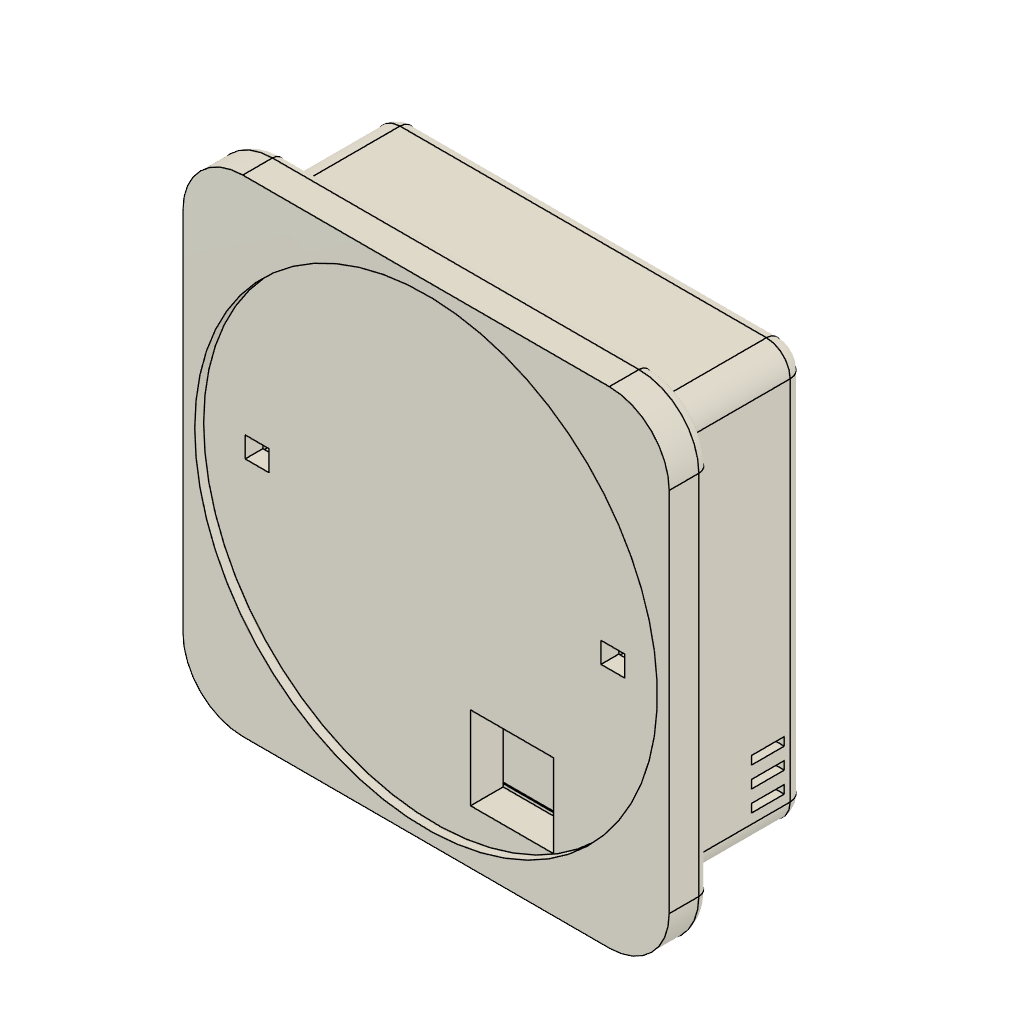
co2_wall_sensor (Autodesk Fusion 360 design; units mm, degrees)
part number: 2026-10-04-22-38-18-043
part number: 2026-10-04-22-38-18-293
part number: 2026-10-04-22-38-22-354
part number: 2026-10-04-22-38-25-106
part number: 2026-10-04-22-38-27-455
part number: 2026-10-04-22-38-30-527
part number: 2026-10-04-22-38-34-110
part number: 2026-10-04-22-38-35-616
part number: 2026-10-04-22-38-36-232
Autodesk Fusion 360 part; units mm, degrees
ref_plane "Arbeitsebene1" through (0, 0, 11) normal (0, 0, 1) x (1, 0, 0) in component "Housing"
sketch "Skizze1" plane through (0, 0, 11) normal (0, 0, 1) x (1, 0, 0) in component "Housing"
  line L0 (-34.9, -34.9) -> (34.9, -34.9)
  line L1 (34.9, -34.9) -> (34.9, 34.9)
  line L2 (34.9, 34.9) -> (-34.9, 34.9)
  line L3 (-34.9, 34.9) -> (-34.9, -34.9)
extrude "BaseBody (1)" add sketch "Skizze1" along normal mid plane 22 makes body 1 in component "Housing"
fillet "CornerRadius" radius 4 4 edges at (-34.9, 34.9, 11) (34.9, 34.9, 11) (34.9, -34.9, 11) (-34.9, -34.9, 11) on bodies 1 in component "Housing"
fillet "SoftFrontEdge" radius 2.5 64 edges at (-33.7284, -33.7284, 0) (0, -34.9, 0) (33.7284, -33.7284, 0) (34.9, 0, 0) (33.7284, 33.7284, 0) (0, 34.9, 0) (-33.7284, 33.7284, 0) (-34.9, 0, 0) (-34.9, 0, 0) (-33.7284, 33.7284, 0) (0, 34.9, 0) (33.7284, 33.7284, 0) (34.9, 0, 0) (33.7284, -33.7284, 0) (0, -34.9, 0) (-33.7284, -33.7284, 0) (-33.7284, 33.7284, 0) (-34.9, 0, 0) (-33.7284, -33.7284, 0) (0, -34.9, 0) (33.7284, -33.7284, 0) (34.9, 0, 0) (33.7284, 33.7284, 0) (0, 34.9, 0) (0, 34.9, 0) (33.7284, 33.7284, 0) (34.9, 0, 0) (33.7284, -33.7284, 0) (0, -34.9, 0) (-33.7284, -33.7284, 0) (-34.9, 0, 0) (-33.7284, 33.7284, 0) (33.7284, 33.7284, 0) (0, 34.9, 0) (-33.7284, 33.7284, 0) (-34.9, 0, 0) (-33.7284, -33.7284, 0) (0, -34.9, 0) (33.7284, -33.7284, 0) (34.9, 0, 0) (34.9, 0, 0) (33.7284, -33.7284, 0) (0, -34.9, 0) (-33.7284, -33.7284, 0) (-34.9, 0, 0) (-33.7284, 33.7284, 0) (0, 34.9, 0) (33.7284, 33.7284, 0) (33.7284, -33.7284, 0) (34.9, 0, 0) (33.7284, 33.7284, 0) (0, 34.9, 0) (-33.7284, 33.7284, 0) (-34.9, 0, 0) (-33.7284, -33.7284, 0) (0, -34.9, 0) (0, -34.9, 0) (-33.7284, -33.7284, 0) (-34.9, 0, 0) (-33.7284, 33.7284, 0) (0, 34.9, 0) (33.7284, 33.7284, 0) (34.9, 0, 0) (33.7284, -33.7284, 0) on bodies 1 in component "Housing"
ref_plane "Arbeitsebene2" through (0, 0, 21.25) normal (0, 0, 1) x (1, 0, 0) in component "Housing"
sketch "Skizze2" plane through (0, 0, 21.25) normal (0, 0, 1) x (1, 0, 0) in component "Housing"
  line L0 (-32.9, -32.9) -> (32.9, -32.9)
  line L1 (32.9, -32.9) -> (32.9, 32.9)
  line L2 (32.9, 32.9) -> (-32.9, 32.9)
  line L3 (-32.9, 32.9) -> (-32.9, -32.9)
extrude "CoverSeat (1)" cut sketch "Skizze2" along normal mid plane 3.5 bodies 1 in component "Housing"
ref_plane "Arbeitsebene3" through (0, 0, 11.25) normal (0, 0, 1) x (1, 0, 0) in component "Housing"
sketch "Skizze3" plane through (0, 0, 11.25) normal (0, 0, 1) x (1, 0, 0) in component "Housing"
  line L0 (-31.4, -7.7) -> (27.2, -7.7)
  line L1 (27.2, -7.7) -> (27.2, 27.9)
  line L2 (27.2, 27.9) -> (-31.4, 27.9)
  line L3 (-31.4, 27.9) -> (-31.4, -7.7)
extrude "DisplayBay (1)" cut sketch "Skizze3" along normal mid plane 18.5 bodies 1 in component "Housing"
ref_plane "Arbeitsebene4" through (0, 0, 0.75) normal (0, 0, 1) x (1, 0, 0) in component "Housing"
sketch "Skizze4" plane through (0, 0, 0.75) normal (0, 0, 1) x (1, 0, 0) in component "Housing"
  line L0 (-20.9, -5.7) -> (20.9, -5.7)
  line L1 (20.9, -5.7) -> (20.9, 25.9)
  line L2 (20.9, 25.9) -> (-20.9, 25.9)
  line L3 (-20.9, 25.9) -> (-20.9, -5.7)
extrude "DisplayWindow (1)" cut sketch "Skizze4" along normal mid plane 3.5 bodies 1 in component "Housing"
fillet "WindowCorners" radius 1 4 edges at (20.9, -5.7, 1) (-20.9, -5.7, 1) (-20.9, 25.9, 1) (20.9, 25.9, 1) on bodies 1 in component "Housing"
chamfer "WindowChamfer" distance 0.8 angle 45 8 edges at (0, 25.9, 0) (-20.6071, 25.6071, 0) (-20.9, 10.1, 0) (-20.6071, -5.4071, 0) (0, -5.7, 0) (20.6071, -5.4071, 0) (20.9, 10.1, 0) (20.6071, 25.6071, 0) tangent chain off on bodies 1 in component "Housing"
ref_plane "Arbeitsebene5" through (0, 0, 3.25) normal (0, 0, 1) x (1, 0, 0) in component "Housing"
sketch "Skizze5" plane through (0, 0, 3.25) normal (0, 0, 1) x (1, 0, 0) in component "Housing"
  circle A0 centre (-28.6, -4.9) radius 2.3
  circle A1 centre (-28.6, 25.1) radius 2.3
  circle A2 centre (24.4, -4.9) radius 2.3
  circle A3 centre (24.4, 25.1) radius 2.3
extrude "LcdBosses (1)" add sketch "Skizze5" along normal mid plane 2.5 bodies 1 in component "Housing"
ref_plane "Arbeitsebene6" through (0, 0, 2.85) normal (0, 0, 1) x (1, 0, 0) in component "Housing"
sketch "Skizze6" plane through (0, 0, 2.85) normal (0, 0, 1) x (1, 0, 0) in component "Housing"
  circle A0 centre (-28.6, -4.9) radius 1.5
  circle A1 centre (-28.6, 25.1) radius 1.5
  circle A2 centre (24.4, -4.9) radius 1.5
  circle A3 centre (24.4, 25.1) radius 1.5
extrude "M2InsertHoles (1)" cut sketch "Skizze6" along normal mid plane 3.5 bodies 1 in component "Housing"
ref_plane "Arbeitsebene7" through (0, 0, 11.25) normal (0, 0, 1) x (1, 0, 0) in component "Housing"
sketch "Skizze7" plane through (0, 0, 11.25) normal (0, 0, 1) x (1, 0, 0) in component "Housing"
  line L0 (-32.9, -32.9) -> (32.9, -32.9)
  line L1 (32.9, -32.9) -> (32.9, -10.2)
  line L2 (32.9, -10.2) -> (-32.9, -10.2)
  line L3 (-32.9, -10.2) -> (-32.9, -32.9)
extrude "Chin (1)" cut sketch "Skizze7" along normal mid plane 18.5 bodies 1 in component "Housing"
ref_plane "Arbeitsebene8" through (0, 0, 16.75) normal (0, 0, 1) x (1, 0, 0) in component "Housing"
sketch "Skizze8" plane through (0, 0, 16.75) normal (0, 0, 1) x (1, 0, 0) in component "Housing"
  line L0 (3, -10.7) -> (23, -10.7)
  line L1 (23, -10.7) -> (23, -7.2)
  line L2 (23, -7.2) -> (3, -7.2)
  line L3 (3, -7.2) -> (3, -10.7)
extrude "EspPassage (1)" cut sketch "Skizze8" along normal mid plane 7.5 bodies 1 in component "Housing"
ref_plane "Arbeitsebene9" through (0, 0, 10.75) normal (0, 0, 1) x (1, 0, 0) in component "Housing"
sketch "Skizze9" plane through (0, 0, 10.75) normal (0, 0, 1) x (1, 0, 0) in component "Housing"
  circle A0 centre (-30.5, -30.5) radius 2.5
  circle A1 centre (30.5, -30.5) radius 2.5
extrude "CoverBossesBottom (1)" add sketch "Skizze9" along normal mid plane 17.5 bodies 1 in component "Housing"
ref_plane "Arbeitsebene10" through (0, 0, 6.5) normal (0, 0, 1) x (1, 0, 0) in component "Housing"
sketch "Skizze10" plane through (0, 0, 6.5) normal (0, 0, 1) x (1, 0, 0) in component "Housing"
  circle A0 centre (-30.5, -12.6) radius 2.5
  circle A1 centre (30.5, -12.6) radius 2.5
extrude "CarrierBosses (1)" add sketch "Skizze10" along normal mid plane 9 bodies 1 in component "Housing"
ref_plane "Arbeitsebene11" through (0, 0, 17.85) normal (0, 0, 1) x (1, 0, 0) in component "Housing"
sketch "Skizze11" plane through (0, 0, 17.85) normal (0, 0, 1) x (1, 0, 0) in component "Housing"
  circle A0 centre (-30.5, -30.5) radius 1.5
  circle A1 centre (30.5, -30.5) radius 1.5
  circle A2 centre (-20, 30.4) radius 1.5
  circle A3 centre (20, 30.4) radius 1.5
extrude "M2InsertHoles (2)" cut sketch "Skizze11" along normal mid plane 3.5 bodies 1 in component "Housing"
ref_plane "Arbeitsebene12" through (0, 0, 9.35) normal (0, 0, 1) x (1, 0, 0) in component "Housing"
sketch "Skizze12" plane through (0, 0, 9.35) normal (0, 0, 1) x (1, 0, 0) in component "Housing"
  circle A0 centre (-30.5, -12.6) radius 1.5
  circle A1 centre (30.5, -12.6) radius 1.5
extrude "M2InsertHoles (3)" cut sketch "Skizze12" along normal mid plane 3.5 bodies 1 in component "Housing"
ref_plane "Arbeitsebene13" through (0, 0, 10.25) normal (0, 0, 1) x (1, 0, 0) in component "Housing"
sketch "Skizze13" plane through (0, 0, 10.25) normal (0, 0, 1) x (1, 0, 0) in component "Housing"
  line L0 (-32.9, -32.9) -> (-31.7, -32.9)
  line L1 (-31.7, -32.9) -> (-31.7, -10.2)
  line L2 (-31.7, -10.2) -> (-32.9, -10.2)
  line L3 (-32.9, -10.2) -> (-32.9, -32.9)
extrude "CarrierLedge (1)" add sketch "Skizze13" along normal mid plane 1.5 bodies 1 in component "Housing"
ref_plane "Arbeitsebene14" through (0, 0, 10.25) normal (0, 0, 1) x (1, 0, 0) in component "Housing"
sketch "Skizze14" plane through (0, 0, 10.25) normal (0, 0, 1) x (1, 0, 0) in component "Housing"
  line L0 (31.7, -32.9) -> (32.9, -32.9)
  line L1 (32.9, -32.9) -> (32.9, -10.2)
  line L2 (32.9, -10.2) -> (31.7, -10.2)
  line L3 (31.7, -10.2) -> (31.7, -32.9)
extrude "CarrierLedge (2)" add sketch "Skizze14" along normal mid plane 1.5 bodies 1 in component "Housing"
ref_plane "Arbeitsebene15" through (0, -33.9, 0) normal (0, 1, 0) x (0, 0, 1) in component "Housing"
sketch "Skizze15" plane through (0, -33.9, 0) normal (0, 1, 0) x (1, 0, 0) in component "Housing"
  line L0 (-21.7, -3.5) -> (-20.3, -3.5)
  line L1 (-20.3, -3.5) -> (-20.3, -9)
  line L2 (-20.3, -9) -> (-21.7, -9)
  line L3 (-21.7, -9) -> (-21.7, -3.5)
  line L4 (-18.2, -3.5) -> (-16.8, -3.5)
  line L5 (-16.8, -3.5) -> (-16.8, -9)
  line L6 (-16.8, -9) -> (-18.2, -9)
  line L7 (-18.2, -9) -> (-18.2, -3.5)
  line L8 (-14.7, -3.5) -> (-13.3, -3.5)
  line L9 (-13.3, -3.5) -> (-13.3, -9)
  line L10 (-13.3, -9) -> (-14.7, -9)
  line L11 (-14.7, -9) -> (-14.7, -3.5)
  line L12 (-11.2, -3.5) -> (-9.8, -3.5)
  line L13 (-9.8, -3.5) -> (-9.8, -9)
  line L14 (-9.8, -9) -> (-11.2, -9)
  line L15 (-11.2, -9) -> (-11.2, -3.5)
  line L16 (-7.7, -3.5) -> (-6.3, -3.5)
  line L17 (-6.3, -3.5) -> (-6.3, -9)
  line L18 (-6.3, -9) -> (-7.7, -9)
  line L19 (-7.7, -9) -> (-7.7, -3.5)
  line L20 (-4.2, -3.5) -> (-2.8, -3.5)
  line L21 (-2.8, -3.5) -> (-2.8, -9)
  line L22 (-2.8, -9) -> (-4.2, -9)
  line L23 (-4.2, -9) -> (-4.2, -3.5)
  line L24 (-0.7, -3.5) -> (0.7, -3.5)
  line L25 (0.7, -3.5) -> (0.7, -9)
  line L26 (0.7, -9) -> (-0.7, -9)
  line L27 (-0.7, -9) -> (-0.7, -3.5)
  line L28 (2.8, -3.5) -> (4.2, -3.5)
  line L29 (4.2, -3.5) -> (4.2, -9)
  line L30 (4.2, -9) -> (2.8, -9)
  line L31 (2.8, -9) -> (2.8, -3.5)
  line L32 (6.3, -3.5) -> (7.7, -3.5)
  line L33 (7.7, -3.5) -> (7.7, -9)
  line L34 (7.7, -9) -> (6.3, -9)
  line L35 (6.3, -9) -> (6.3, -3.5)
  line L36 (9.8, -3.5) -> (11.2, -3.5)
  line L37 (11.2, -3.5) -> (11.2, -9)
  line L38 (11.2, -9) -> (9.8, -9)
  line L39 (9.8, -9) -> (9.8, -3.5)
  line L40 (13.3, -3.5) -> (14.7, -3.5)
  line L41 (14.7, -3.5) -> (14.7, -9)
  line L42 (14.7, -9) -> (13.3, -9)
  line L43 (13.3, -9) -> (13.3, -3.5)
  line L44 (16.8, -3.5) -> (18.2, -3.5)
  line L45 (18.2, -3.5) -> (18.2, -9)
  line L46 (18.2, -9) -> (16.8, -9)
  line L47 (16.8, -9) -> (16.8, -3.5)
  line L48 (20.3, -3.5) -> (21.7, -3.5)
  line L49 (21.7, -3.5) -> (21.7, -9)
  line L50 (21.7, -9) -> (20.3, -9)
  line L51 (20.3, -9) -> (20.3, -3.5)
extrude "BottomVents (1)" cut sketch "Skizze15" along normal mid plane 3 bodies 1 in component "Housing"
ref_plane "Arbeitsebene16" through (-33.9, 0, 0) normal (1, 0, 0) x (0, 1, 0) in component "Housing"
sketch "Skizze16" plane through (-33.9, 0, 0) normal (1, 0, 0) x (0, 0, -1) in component "Housing"
  line L0 (-3.5, -29.25) -> (-9, -29.25)
  line L1 (-9, -29.25) -> (-9, -27.85)
  line L2 (-9, -27.85) -> (-3.5, -27.85)
  line L3 (-3.5, -27.85) -> (-3.5, -29.25)
  line L4 (-3.5, -25.75) -> (-9, -25.75)
  line L5 (-9, -25.75) -> (-9, -24.35)
  line L6 (-9, -24.35) -> (-3.5, -24.35)
  line L7 (-3.5, -24.35) -> (-3.5, -25.75)
  line L8 (-3.5, -22.25) -> (-9, -22.25)
  line L9 (-9, -22.25) -> (-9, -20.85)
  line L10 (-9, -20.85) -> (-3.5, -20.85)
  line L11 (-3.5, -20.85) -> (-3.5, -22.25)
extrude "SideVents (1)" cut sketch "Skizze16" along normal mid plane 3 bodies 1 in component "Housing"
ref_plane "Arbeitsebene17" through (33.9, 0, 0) normal (1, 0, 0) x (0, 1, 0) in component "Housing"
sketch "Skizze17" plane through (33.9, 0, 0) normal (1, 0, 0) x (0, 0, -1) in component "Housing"
  line L0 (-3.5, -29.25) -> (-9, -29.25)
  line L1 (-9, -29.25) -> (-9, -27.85)
  line L2 (-9, -27.85) -> (-3.5, -27.85)
  line L3 (-3.5, -27.85) -> (-3.5, -29.25)
  line L4 (-3.5, -25.75) -> (-9, -25.75)
  line L5 (-9, -25.75) -> (-9, -24.35)
  line L6 (-9, -24.35) -> (-3.5, -24.35)
  line L7 (-3.5, -24.35) -> (-3.5, -25.75)
  line L8 (-3.5, -22.25) -> (-9, -22.25)
  line L9 (-9, -22.25) -> (-9, -20.85)
  line L10 (-9, -20.85) -> (-3.5, -20.85)
  line L11 (-3.5, -20.85) -> (-3.5, -22.25)
extrude "SideVents (2)" cut sketch "Skizze17" along normal mid plane 3 bodies 1 in component "Housing"
ref_plane "Arbeitsebene18" through (0, 0, 16.1) normal (0, 0, 1) x (1, 0, 0) in component "Housing"
sketch "Skizze18" plane through (0, 0, 16.1) normal (0, 0, 1) x (1, 0, 0) in component "Housing"
  line L0 (6.5, -35.9) -> (19.5, -35.9)
  line L1 (19.5, -35.9) -> (19.5, -32.8)
  line L2 (19.5, -32.8) -> (6.5, -32.8)
  line L3 (6.5, -32.8) -> (6.5, -35.9)
extrude "BottomCableOpening (1)" cut sketch "Skizze18" along normal mid plane 6.6 bodies 1 in component "Housing"
ref_plane "Arbeitsebene19" through (0, 0, 16.1) normal (0, 0, 1) x (1, 0, 0) in component "Housing"
sketch "Skizze19" plane through (0, 0, 16.1) normal (0, 0, 1) x (1, 0, 0) in component "Housing"
  line L0 (6.5, -34.9) -> (19.5, -34.9)
  line L1 (19.5, -34.9) -> (19.5, -34.3)
  line L2 (19.5, -34.3) -> (6.5, -34.3)
  line L3 (6.5, -34.3) -> (6.5, -34.9)
extrude "BottomKnockout (1)" add sketch "Skizze19" along normal mid plane 6.6 bodies 1 in component "Housing"
ref_plane "Arbeitsebene1" through (0, 0, 12) normal (0, 0, 1) x (1, 0, 0) in component "SensorCarrier"
sketch "Skizze1 (2)" plane through (0, 0, 12) normal (0, 0, 1) x (1, 0, 0) in component "SensorCarrier"
  line L0 (-32.7, -32.7) -> (32.7, -32.7)
  line L1 (32.7, -32.7) -> (32.7, -10.4)
  line L2 (32.7, -10.4) -> (-32.7, -10.4)
  line L3 (-32.7, -10.4) -> (-32.7, -32.7)
extrude "Carrier (1)" add sketch "Skizze1 (2)" along normal mid plane 2 separate body makes body 2 in component "SensorCarrier"
ref_plane "Arbeitsebene2" through (0, 0, 12) normal (0, 0, 1) x (1, 0, 0) in component "SensorCarrier"
sketch "Skizze2 (2)" plane through (0, 0, 12) normal (0, 0, 1) x (1, 0, 0) in component "SensorCarrier"
  line L0 (-33.3, -35.3) -> (-27.7, -35.3)
  line L1 (-27.7, -35.3) -> (-27.7, -27.7)
  line L2 (-27.7, -27.7) -> (-33.3, -27.7)
  line L3 (-33.3, -27.7) -> (-33.3, -35.3)
extrude "BossNotch (1)" cut sketch "Skizze2 (2)" along normal mid plane 4 bodies 2 in component "SensorCarrier"
ref_plane "Arbeitsebene3" through (0, 0, 12) normal (0, 0, 1) x (1, 0, 0) in component "SensorCarrier"
sketch "Skizze3 (2)" plane through (0, 0, 12) normal (0, 0, 1) x (1, 0, 0) in component "SensorCarrier"
  line L0 (27.7, -35.3) -> (33.3, -35.3)
  line L1 (33.3, -35.3) -> (33.3, -27.7)
  line L2 (33.3, -27.7) -> (27.7, -27.7)
  line L3 (27.7, -27.7) -> (27.7, -35.3)
extrude "BossNotch (2)" cut sketch "Skizze3 (2)" along normal mid plane 4 bodies 2 in component "SensorCarrier"
ref_plane "Arbeitsebene4" through (0, 0, 8.05) normal (0, 0, 1) x (1, 0, 0) in component "SensorCarrier"
sketch "Skizze4 (2)" plane through (0, 0, 8.05) normal (0, 0, 1) x (1, 0, 0) in component "SensorCarrier"
  circle A0 centre (-30.5, -12.6) radius 1.2
  circle A1 centre (30.5, -12.6) radius 1.2
extrude "M2Clearance (1)" cut sketch "Skizze4 (2)" along normal mid plane 10.1 bodies 2 in component "SensorCarrier"
ref_plane "Arbeitsebene5" through (0, 0, 10.25) normal (0, 0, 1) x (1, 0, 0) in component "SensorCarrier"
sketch "Skizze5 (2)" plane through (0, 0, 10.25) normal (0, 0, 1) x (1, 0, 0) in component "SensorCarrier"
  line L0 (-11.5, -31.85) -> (-10.3, -31.85)
  line L1 (-10.3, -31.85) -> (-10.3, -11.25)
  line L2 (-10.3, -11.25) -> (-11.5, -11.25)
  line L3 (-11.5, -11.25) -> (-11.5, -31.85)
extrude "ScdGuide (1)" add sketch "Skizze5 (2)" along normal mid plane 1.5 bodies 2 in component "SensorCarrier"
ref_plane "Arbeitsebene6" through (0, 0, 10.25) normal (0, 0, 1) x (1, 0, 0) in component "SensorCarrier"
sketch "Skizze6 (2)" plane through (0, 0, 10.25) normal (0, 0, 1) x (1, 0, 0) in component "SensorCarrier"
  line L0 (10.3, -31.85) -> (11.5, -31.85)
  line L1 (11.5, -31.85) -> (11.5, -11.25)
  line L2 (11.5, -11.25) -> (10.3, -11.25)
  line L3 (10.3, -11.25) -> (10.3, -31.85)
extrude "ScdGuide (2)" add sketch "Skizze6 (2)" along normal mid plane 1.5 bodies 2 in component "SensorCarrier"
ref_plane "Arbeitsebene7" through (0, 0, 12) normal (0, 0, 1) x (1, 0, 0) in component "SensorCarrier"
sketch "Skizze7 (2)" plane through (0, 0, 12) normal (0, 0, 1) x (1, 0, 0) in component "SensorCarrier"
  line L0 (-16, -14.2) -> (-12, -14.2)
  line L1 (-12, -14.2) -> (-12, -10.1)
  line L2 (-12, -10.1) -> (-16, -10.1)
  line L3 (-16, -10.1) -> (-16, -14.2)
extrude "ScdCableNotch (1)" cut sketch "Skizze7 (2)" along normal mid plane 3 bodies 2 in component "SensorCarrier"
ref_plane "Arbeitsebene8" through (0, 0, 13.25) normal (0, 0, 1) x (1, 0, 0) in component "SensorCarrier"
sketch "Skizze8 (2)" plane through (0, 0, 13.25) normal (0, 0, 1) x (1, 0, 0) in component "SensorCarrier"
  line L0 (6.25, -19.9) -> (7.75, -19.9)
  line L1 (7.75, -19.9) -> (7.75, -10.4)
  line L2 (7.75, -10.4) -> (6.25, -10.4)
  line L3 (6.25, -10.4) -> (6.25, -19.9)
extrude "C3Rib (1)" add sketch "Skizze8 (2)" along normal mid plane 0.5 bodies 2 in component "SensorCarrier"
ref_plane "Arbeitsebene9" through (0, 0, 13.25) normal (0, 0, 1) x (1, 0, 0) in component "SensorCarrier"
sketch "Skizze9 (2)" plane through (0, 0, 13.25) normal (0, 0, 1) x (1, 0, 0) in component "SensorCarrier"
  line L0 (18.25, -19.9) -> (19.75, -19.9)
  line L1 (19.75, -19.9) -> (19.75, -10.4)
  line L2 (19.75, -10.4) -> (18.25, -10.4)
  line L3 (18.25, -10.4) -> (18.25, -19.9)
extrude "C3Rib (2)" add sketch "Skizze9 (2)" along normal mid plane 0.5 bodies 2 in component "SensorCarrier"
ref_plane "Arbeitsebene10" through (0, 0, 14.25) normal (0, 0, 1) x (1, 0, 0) in component "SensorCarrier"
sketch "Skizze10 (2)" plane through (0, 0, 14.25) normal (0, 0, 1) x (1, 0, 0) in component "SensorCarrier"
  line L0 (2.6, -19.9) -> (3.8, -19.9)
  line L1 (3.8, -19.9) -> (3.8, -11.9)
  line L2 (3.8, -11.9) -> (2.6, -11.9)
  line L3 (2.6, -11.9) -> (2.6, -19.9)
extrude "C3SideGuide (1)" add sketch "Skizze10 (2)" along normal mid plane 2.5 bodies 2 in component "SensorCarrier"
ref_plane "Arbeitsebene11" through (0, 0, 14.25) normal (0, 0, 1) x (1, 0, 0) in component "SensorCarrier"
sketch "Skizze11 (2)" plane through (0, 0, 14.25) normal (0, 0, 1) x (1, 0, 0) in component "SensorCarrier"
  line L0 (22.2, -19.9) -> (23.4, -19.9)
  line L1 (23.4, -19.9) -> (23.4, -11.9)
  line L2 (23.4, -11.9) -> (22.2, -11.9)
  line L3 (22.2, -11.9) -> (22.2, -19.9)
extrude "C3SideGuide (2)" add sketch "Skizze11 (2)" along normal mid plane 2.5 bodies 2 in component "SensorCarrier"
ref_plane "Arbeitsebene1" through (0, 0, 20.75) normal (0, 0, 1) x (1, 0, 0) in component "BackCover"
sketch "Skizze1 (3)" plane through (0, 0, 20.75) normal (0, 0, 1) x (1, 0, 0) in component "BackCover"
  line L0 (-32.7, -32.7) -> (32.7, -32.7)
  line L1 (32.7, -32.7) -> (32.7, 32.7)
  line L2 (32.7, 32.7) -> (-32.7, 32.7)
  line L3 (-32.7, 32.7) -> (-32.7, -32.7)
extrude "Cover (1)" add sketch "Skizze1 (3)" along normal mid plane 2.5 separate body makes body 3 in component "BackCover"
ref_plane "Arbeitsebene2" through (0, 0, 17.05) normal (0, 0, 1) x (1, 0, 0) in component "BackCover"
sketch "Skizze2 (3)" plane through (0, 0, 17.05) normal (0, 0, 1) x (1, 0, 0) in component "BackCover"
  circle A0 centre (-30.5, -30.5) radius 1.2
  circle A1 centre (30.5, -30.5) radius 1.2
  circle A2 centre (-20, 30.4) radius 1.2
  circle A3 centre (20, 30.4) radius 1.2
extrude "M2Clearance (1)'" cut sketch "Skizze2 (3)" along normal mid plane 10.1 bodies 3 in component "BackCover"
ref_plane "Arbeitsebene3" through (0, 0, 21.4) normal (0, 0, 1) x (1, 0, 0) in component "BackCover"
sketch "Skizze3 (3)" plane through (0, 0, 21.4) normal (0, 0, 1) x (1, 0, 0) in component "BackCover"
  circle A0 centre (-30.5, -30.5) radius 2.1
  circle A1 centre (30.5, -30.5) radius 2.1
  circle A2 centre (-20, 30.4) radius 2.1
  circle A3 centre (20, 30.4) radius 2.1
extrude "M2HeadRecess (1)" cut sketch "Skizze3 (3)" along normal mid plane 1.4 bodies 3 in component "BackCover"
ref_plane "Arbeitsebene4" through (0, 0, 20.75) normal (0, 0, 1) x (1, 0, 0) in component "BackCover"
sketch "Skizze4 (3)" plane through (0, 0, 20.75) normal (0, 0, 1) x (1, 0, 0) in component "BackCover"
  line L0 (6, -32.4) -> (20, -32.4)
  line L1 (20, -32.4) -> (20, -20.4)
  line L2 (20, -20.4) -> (6, -20.4)
  line L3 (6, -20.4) -> (6, -32.4)
extrude "BackCableOpening (1)" cut sketch "Skizze4 (3)" along normal mid plane 4.5 bodies 3 in component "BackCover"
ref_plane "Arbeitsebene5" through (0, 0, 21.7) normal (0, 0, 1) x (1, 0, 0) in component "BackCover"
sketch "Skizze5 (3)" plane through (0, 0, 21.7) normal (0, 0, 1) x (1, 0, 0) in component "BackCover"
  line L0 (6, -32.4) -> (20, -32.4)
  line L1 (20, -32.4) -> (20, -20.4)
  line L2 (20, -20.4) -> (6, -20.4)
  line L3 (6, -20.4) -> (6, -32.4)
extrude "BackKnockout (1)" add sketch "Skizze5 (3)" along normal mid plane 0.6 bodies 3 in component "BackCover"
ref_plane "Arbeitsebene6" through (0, -3, 0) normal (0, 1, 0) x (0, 0, 1) in component "BackCover"
sketch "Skizze6 (3)" plane through (0, -3, 0) normal (0, 1, 0) x (1, 0, 0) in component "BackCover"
  line L0 (-6, -22) -> (6, -22)
  line L1 (6, -22) -> (8, -25)
  line L2 (8, -25) -> (-8, -25)
  line L3 (-8, -25) -> (-6, -22)
extrude "Rail (1)" add sketch "Skizze6 (3)" along normal mid plane 14 bodies 3 in component "BackCover"
ref_plane "Arbeitsebene1" through (0, 0, 25.5) normal (0, 0, 1) x (1, 0, 0) in component "WallPlate"
sketch "Skizze1 (4)" plane through (0, 0, 25.5) normal (0, 0, 1) x (1, 0, 0) in component "WallPlate"
  line L0 (-41, -41) -> (41, -41)
  line L1 (41, -41) -> (41, 41)
  line L2 (41, 41) -> (-41, 41)
  line L3 (-41, 41) -> (-41, -41)
extrude "Plate (1)" add sketch "Skizze1 (4)" along normal mid plane 7 separate body makes body 4 in component "WallPlate"
fillet "ConcentricCorners" radius 10.1 4 edges at (-41, 41, 25.5) (41, 41, 25.5) (41, -41, 25.5) (-41, -41, 25.5) on bodies 4 in component "WallPlate"
fillet "FrontEdge" radius 2 64 edges at (-38.0418, -38.0418, 22) (0, -41, 22) (38.0418, -38.0418, 22) (41, 0, 22) (38.0418, 38.0418, 22) (0, 41, 22) (-38.0418, 38.0418, 22) (-41, 0, 22) (-41, 0, 22) (-38.0418, 38.0418, 22) (0, 41, 22) (38.0418, 38.0418, 22) (41, 0, 22) (38.0418, -38.0418, 22) (0, -41, 22) (-38.0418, -38.0418, 22) (-38.0418, 38.0418, 22) (-41, 0, 22) (-38.0418, -38.0418, 22) (0, -41, 22) (38.0418, -38.0418, 22) (41, 0, 22) (38.0418, 38.0418, 22) (0, 41, 22) (0, 41, 22) (38.0418, 38.0418, 22) (41, 0, 22) (38.0418, -38.0418, 22) (0, -41, 22) (-38.0418, -38.0418, 22) (-41, 0, 22) (-38.0418, 38.0418, 22) (38.0418, 38.0418, 22) (0, 41, 22) (-38.0418, 38.0418, 22) (-41, 0, 22) (-38.0418, -38.0418, 22) (0, -41, 22) (38.0418, -38.0418, 22) (41, 0, 22) (41, 0, 22) (38.0418, -38.0418, 22) (0, -41, 22) (-38.0418, -38.0418, 22) (-41, 0, 22) (-38.0418, 38.0418, 22) (0, 41, 22) (38.0418, 38.0418, 22) (38.0418, -38.0418, 22) (41, 0, 22) (38.0418, 38.0418, 22) (0, 41, 22) (-38.0418, 38.0418, 22) (-41, 0, 22) (-38.0418, -38.0418, 22) (0, -41, 22) (0, -41, 22) (-38.0418, -38.0418, 22) (-41, 0, 22) (-38.0418, 38.0418, 22) (0, 41, 22) (38.0418, 38.0418, 22) (41, 0, 22) (38.0418, -38.0418, 22) on bodies 4 in component "WallPlate"
ref_plane "Arbeitsebene2" through (0, 0, 28.75) normal (0, 0, 1) x (1, 0, 0) in component "WallPlate"
sketch "Skizze2 (4)" plane through (0, 0, 28.75) normal (0, 0, 1) x (1, 0, 0) in component "WallPlate"
  circle A0 centre (0, 0) radius 39
extrude "BoxRimRecess (1)" cut sketch "Skizze2 (4)" along normal mid plane 2.5 bodies 4 in component "WallPlate"
ref_plane "Arbeitsebene3" through (0, -3, 0) normal (0, 1, 0) x (0, 0, 1) in component "WallPlate"
sketch "Skizze3 (4)" plane through (0, -3, 0) normal (0, 1, 0) x (1, 0, 0) in component "WallPlate"
  line L0 (-6.3, -21.99) -> (6.3, -21.99)
  line L1 (6.3, -21.99) -> (8.3, -25.29)
  line L2 (8.3, -25.29) -> (-8.3, -25.29)
  line L3 (-8.3, -25.29) -> (-6.3, -21.99)
extrude "DovetailSlot (1)" cut sketch "Skizze3 (4)" along normal mid plane 14.6 bodies 4 in component "WallPlate"
ref_plane "Arbeitsebene4" through (0, 0, 23.645) normal (0, 0, 1) x (1, 0, 0) in component "WallPlate"
sketch "Skizze4 (4)" plane through (0, 0, 23.645) normal (0, 0, 1) x (1, 0, 0) in component "WallPlate"
  line L0 (-8.3, 4.29) -> (8.3, 4.29)
  line L1 (8.3, 4.29) -> (8.3, 19.3)
  line L2 (8.3, 19.3) -> (-8.3, 19.3)
  line L3 (-8.3, 19.3) -> (-8.3, 4.29)
extrude "InsertionWindow (1)" cut sketch "Skizze4 (4)" along normal mid plane 3.31 bodies 4 in component "WallPlate"
ref_plane "Arbeitsebene5" through (0, 0, 25.5) normal (0, 0, 1) x (1, 0, 0) in component "WallPlate"
sketch "Skizze5 (4)" plane through (0, 0, 25.5) normal (0, 0, 1) x (1, 0, 0) in component "WallPlate"
  line L0 (6, -33.4) -> (20, -33.4)
  line L1 (20, -33.4) -> (20, -19.4)
  line L2 (20, -19.4) -> (6, -19.4)
  line L3 (6, -19.4) -> (6, -33.4)
extrude "CablePassage (1)" cut sketch "Skizze5 (4)" along normal mid plane 9 bodies 4 in component "WallPlate"
ref_plane "Arbeitsebene6" through (0, 0, 25.5) normal (0, 0, 1) x (1, 0, 0) in component "WallPlate"
sketch "Skizze6 (4)" plane through (0, 0, 25.5) normal (0, 0, 1) x (1, 0, 0) in component "WallPlate"
  line L0 (-32, -1.75) -> (-28, -1.75)
  line L1 (-28, -1.75) -> (-28, 1.75)
  line L2 (-28, 1.75) -> (-32, 1.75)
  line L3 (-32, 1.75) -> (-32, -1.75)
  line L4 (28, -1.75) -> (32, -1.75)
  line L5 (32, -1.75) -> (32, 1.75)
  line L6 (32, 1.75) -> (28, 1.75)
  line L7 (28, 1.75) -> (28, -1.75)
extrude "ScrewSlots (1)" cut sketch "Skizze6 (4)" along normal mid plane 8 bodies 4 in component "WallPlate"
ref_plane "Arbeitsebene7" through (0, 0, 23) normal (0, 0, 1) x (1, 0, 0) in component "WallPlate"
sketch "Skizze7 (3)" plane through (0, 0, 23) normal (0, 0, 1) x (1, 0, 0) in component "WallPlate"
  line L0 (-33.3, -3.3) -> (-26.7, -3.3)
  line L1 (-26.7, -3.3) -> (-26.7, 3.3)
  line L2 (-26.7, 3.3) -> (-33.3, 3.3)
  line L3 (-33.3, 3.3) -> (-33.3, -3.3)
  line L4 (26.7, -3.3) -> (33.3, -3.3)
  line L5 (33.3, -3.3) -> (33.3, 3.3)
  line L6 (33.3, 3.3) -> (26.7, 3.3)
  line L7 (26.7, 3.3) -> (26.7, -3.3)
extrude "ScrewHeadRecess (1)" cut sketch "Skizze7 (3)" along normal mid plane 3 bodies 4 in component "WallPlate"
ref_plane "Arbeitsebene1" through (0, 0, 0) normal (1, 0, 0) x (0, 1, 0) in component "DeskStand"
sketch "Skizze1 (5)" plane through (0, 0, 0) normal (1, 0, 0) x (0, 0, -1) in component "DeskStand"
  line L0 (2, -45.0014) -> (-46, -34.7986)
  line L1 (-46, -34.7986) -> (-46, -38.7986)
  line L2 (-46, -38.7986) -> (2, -49.0014)
  line L3 (2, -49.0014) -> (2, -45.0014)
extrude "Foot (1)" add sketch "Skizze1 (5)" along normal mid plane 61.8 separate body makes body 5 in component "DeskStand"
ref_plane "Arbeitsebene2" through (0, 0, 0) normal (1, 0, 0) x (0, 1, 0) in component "DeskStand"
sketch "Skizze2 (5)" plane through (0, 0, 0) normal (1, 0, 0) x (0, 0, -1) in component "DeskStand"
  line L0 (-22, -41.9) -> (-22, 23)
  line L1 (-22, 23) -> (-29, 23)
  line L2 (-29, 23) -> (-29, -40.4121)
  line L3 (-29, -40.4121) -> (-22, -41.9)
extrude "Spine (1)" add sketch "Skizze2 (5)" along normal mid plane 28 bodies 5 in component "DeskStand"
ref_plane "Arbeitsebene3" through (0, 0, 0) normal (1, 0, 0) x (0, 1, 0) in component "DeskStand"
sketch "Skizze3 (5)" plane through (0, 0, 0) normal (1, 0, 0) x (0, 0, -1) in component "DeskStand"
  line L0 (-29, -39.4121) -> (-29, 11)
  line L1 (-29, 11) -> (-46, -35.7986)
  line L2 (-46, -35.7986) -> (-29, -39.4121)
extrude "SupportRib (1)" add sketch "Skizze3 (5)" along normal mid plane 3 bodies 5 in component "DeskStand"
ref_plane "Arbeitsebene4" through (0, -3, 0) normal (0, 1, 0) x (0, 0, 1) in component "DeskStand"
sketch "Skizze4 (5)" plane through (0, -3, 0) normal (0, 1, 0) x (1, 0, 0) in component "DeskStand"
  line L0 (-6.3, -21.99) -> (6.3, -21.99)
  line L1 (6.3, -21.99) -> (8.3, -25.29)
  line L2 (8.3, -25.29) -> (-8.3, -25.29)
  line L3 (-8.3, -25.29) -> (-6.3, -21.99)
extrude "DovetailSlot (1)'" cut sketch "Skizze4 (5)" along normal mid plane 14.6 bodies 5 in component "DeskStand"
ref_plane "Arbeitsebene5" through (0, 0, 23.645) normal (0, 0, 1) x (1, 0, 0) in component "DeskStand"
sketch "Skizze5 (5)" plane through (0, 0, 23.645) normal (0, 0, 1) x (1, 0, 0) in component "DeskStand"
  line L0 (-8.3, 4.29) -> (8.3, 4.29)
  line L1 (8.3, 4.29) -> (8.3, 19.3)
  line L2 (8.3, 19.3) -> (-8.3, 19.3)
  line L3 (-8.3, 19.3) -> (-8.3, 4.29)
extrude "InsertionWindow (1)'" cut sketch "Skizze5 (5)" along normal mid plane 3.31 bodies 5 in component "DeskStand"
ref_plane "Arbeitsebene6" through (0, 0, 25.5) normal (0, 0, 1) x (1, 0, 0) in component "DeskStand"
sketch "Skizze6 (5)" plane through (0, 0, 25.5) normal (0, 0, 1) x (1, 0, 0) in component "DeskStand"
  line L0 (6, -33.4) -> (20, -33.4)
  line L1 (20, -33.4) -> (20, -19.4)
  line L2 (20, -19.4) -> (6, -19.4)
  line L3 (6, -19.4) -> (6, -33.4)
extrude "CablePassage (1)'" cut sketch "Skizze6 (5)" along normal mid plane 9 bodies 5 in component "DeskStand"
ref_plane "Arbeitsebene7" through (0, 0, 0) normal (1, 0, 0) x (0, 1, 0) in component "DeskStand"
sketch "Skizze7 (4)" plane through (0, 0, 0) normal (1, 0, 0) x (0, 0, -1) in component "DeskStand"
  line L0 (-38, -35.4991) -> (-47, -33.7986)
  line L1 (-47, -33.7986) -> (-47, -39.7986)
  line L2 (-47, -39.7986) -> (-38, -41.4991)
  line L3 (-38, -41.4991) -> (-38, -35.4991)
extrude "CableNotch (1)" cut sketch "Skizze7 (4)" along normal mid plane 8 bodies 5 in component "DeskStand"
fillet "FootEdges" radius 1.5 2 edges at (0, -49.0014, -2) (0, -45.0014, -2) on bodies 5 in component "DeskStand"
ref_plane "Arbeitsebene1" through (0, 0, 3.25) normal (0, 0, 1) x (1, 0, 0) in component "Dummy_LCD_2inch"
sketch "Skizze1 (6)" plane through (0, 0, 3.25) normal (0, 0, 1) x (1, 0, 0) in component "Dummy_LCD_2inch"
  line L0 (-26.1, -7.25) -> (22.1, -7.25)
  line L1 (22.1, -7.25) -> (22.1, 27.45)
  line L2 (22.1, 27.45) -> (-26.1, 27.45)
  line L3 (-26.1, 27.45) -> (-26.1, -7.25)
extrude "Glass (1)" add sketch "Skizze1 (6)" along normal mid plane 2.5 separate body makes body 6 in component "Dummy_LCD_2inch"
ref_plane "Arbeitsebene2" through (0, 0, 5.3) normal (0, 0, 1) x (1, 0, 0) in component "Dummy_LCD_2inch"
sketch "Skizze2 (6)" plane through (0, 0, 5.3) normal (0, 0, 1) x (1, 0, 0) in component "Dummy_LCD_2inch"
  line L0 (-31.1, -7.4) -> (26.9, -7.4)
  line L1 (26.9, -7.4) -> (26.9, 27.6)
  line L2 (26.9, 27.6) -> (-31.1, 27.6)
  line L3 (-31.1, 27.6) -> (-31.1, -7.4)
extrude "Pcb (1)" add sketch "Skizze2 (6)" along normal mid plane 1.6 separate body makes body 7 in component "Dummy_LCD_2inch"
ref_plane "Arbeitsebene3" through (0, 0, 9.1) normal (0, 0, 1) x (1, 0, 0) in component "Dummy_LCD_2inch"
sketch "Skizze3 (6)" plane through (0, 0, 9.1) normal (0, 0, 1) x (1, 0, 0) in component "Dummy_LCD_2inch"
  line L0 (-27.4, 0.1) -> (-21.4, 0.1)
  line L1 (-21.4, 0.1) -> (-21.4, 20.1)
  line L2 (-21.4, 20.1) -> (-27.4, 20.1)
  line L3 (-27.4, 20.1) -> (-27.4, 0.1)
extrude "PH2Connector (1)" add sketch "Skizze3 (6)" along normal mid plane 6 separate body makes body 8 in component "Dummy_LCD_2inch"
ref_plane "Arbeitsebene1" through (0, 0, 6.945) normal (0, 0, 1) x (1, 0, 0) in component "Dummy_SCD41"
sketch "Skizze1 (7)" plane through (0, 0, 6.945) normal (0, 0, 1) x (1, 0, 0) in component "Dummy_SCD41"
  line L0 (-10, -31.55) -> (10, -31.55)
  line L1 (10, -31.55) -> (10, -11.55)
  line L2 (10, -11.55) -> (-10, -11.55)
  line L3 (-10, -11.55) -> (-10, -31.55)
extrude "SCD41 (1)" add sketch "Skizze1 (7)" along normal mid plane 8.09 separate body makes body 9 in component "Dummy_SCD41"
ref_plane "Arbeitsebene1" through (0, 0, 14) normal (0, 0, 1) x (1, 0, 0) in component "Dummy_ESP32_C3"
sketch "Skizze1 (8)" plane through (0, 0, 14) normal (0, 0, 1) x (1, 0, 0) in component "Dummy_ESP32_C3"
  line L0 (4, -19.9) -> (22, -19.9)
  line L1 (22, -19.9) -> (22, 2.6)
  line L2 (22, 2.6) -> (4, 2.6)
  line L3 (4, 2.6) -> (4, -19.9)
extrude "C3Pcb (1)" add sketch "Skizze1 (8)" along normal mid plane 1 separate body makes body 10 in component "Dummy_ESP32_C3"
ref_plane "Arbeitsebene2" through (0, 0, 16.1) normal (0, 0, 1) x (1, 0, 0) in component "Dummy_ESP32_C3"
sketch "Skizze2 (7)" plane through (0, 0, 16.1) normal (0, 0, 1) x (1, 0, 0) in component "Dummy_ESP32_C3"
  line L0 (8.5, -20.4) -> (17.5, -20.4)
  line L1 (17.5, -20.4) -> (17.5, -12.9)
  line L2 (17.5, -12.9) -> (8.5, -12.9)
  line L3 (8.5, -12.9) -> (8.5, -20.4)
extrude "UsbCSocket (1)" add sketch "Skizze2 (7)" along normal mid plane 3.2 separate body makes body 11 in component "Dummy_ESP32_C3"
ref_plane "Arbeitsebene3" through (0, 0, 16.1) normal (0, 0, 1) x (1, 0, 0) in component "Dummy_ESP32_C3"
sketch "Skizze3 (7)" plane through (0, 0, 16.1) normal (0, 0, 1) x (1, 0, 0) in component "Dummy_ESP32_C3"
  line L0 (7, -32.4) -> (19, -32.4)
  line L1 (19, -32.4) -> (19, -20.4)
  line L2 (19, -20.4) -> (7, -20.4)
  line L3 (7, -20.4) -> (7, -32.4)
extrude "RightAnglePlug (1)" add sketch "Skizze3 (7)" along normal mid plane 6 separate body makes body 12 in component "Dummy_ESP32_C3"
component "Housing" placed x (1, 0, 0) y (0, 1, 0) z (0, 0, 1) at (0, 0, 0)
component "SensorCarrier" placed x (1, 0, 0) y (0, 1, 0) z (0, 0, 1) at (0, 0, 0)
component "BackCover" placed x (1, 0, 0) y (0, 1, 0) z (0, 0, 1) at (0, 0, 0)
component "WallPlate" placed x (1, 0, 0) y (0, 1, 0) z (0, 0, 1) at (0, 0, 0)
component "DeskStand" placed x (1, 0, 0) y (0, 1, 0) z (0, 0, 1) at (0, 0, 0)
component "Dummy_LCD_2inch" placed x (1, 0, 0) y (0, 1, 0) z (0, 0, 1) at (0, 0, 0)
component "Dummy_SCD41" placed x (1, 0, 0) y (0, 1, 0) z (0, 0, 1) at (0, 0, 0)
component "Dummy_ESP32_C3" placed x (1, 0, 0) y (0, 1, 0) z (0, 0, 1) at (0, 0, 0)
named bodies: "Housing", "SensorCarrier", "BackCover", "WallPlate", "DeskStand"
